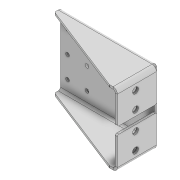
# Autodesk Inventor part: CCM_Mount_A
Saved by Autodesk Inventor 2020 (Build 240168000, 168)
## iProperties
Created: 2021-12-05
Part Number: CCM_Mount_A
Material: 一般
Document SubType Name: Sheet Metal
Designer: ken113
Density: 1 g/cm^3
Sheet Metal Rule: Default_mm
Appearance: 既定
Author: ken113
Autodesk Inventor part; units mm, degrees
ref_plane "YZ Plane" through (0, 0, 0) normal (1, 0, 0) x (0, 1, 0)
ref_plane "XZ Plane" through (0, 0, 0) normal (0, 1, 0) x (-1, 0, 0)
ref_plane "XY Plane" through (0, 0, 0) normal (0, 0, 1) x (1, 0, 0)
sketch "スケッチ1" plane through (0, 0, 0) normal (0, 0, 1) x (1, 0, 0)
  line L0 (-65, -50) -> (65, -50)
  line L1 (65, -50) -> (65, 50)
  line L2 (65, 50) -> (-65, 50)
  line L3 (-65, 50) -> (-65, -50)
  line L4 (-65, -50) -> (65, 50) construction
  line L5 (65, -50) -> (-65, 50) construction
  point P0 (0, 0)
  dimension "d0" = 130
  dimension "d1" = 100
  measures "d0" distance of L1.end L2.end
  measures "d1" distance of L2.end L0.start
extrude "プレート1" add sketch "スケッチ1" along normal blind 3
sketch "スケッチ2" plane through (-65, 47, 0) normal (0, 1, 0) x (-1, 0, 0)
  line L0 (-130, 0) -> (0, 0)
  line L1 (0, 0) -> (0, 60)
  line L2 (0, 60) -> (-130, 60)
  line L3 (-130, 60) -> (-130, 0)
  constraints: 6 end point, 1 horizontal, 1 perpendicular, 1 vertical
edge flange "フランジ1" height 60 angle 90 thickness 3 bend radius 3 thickness toward (0, 1, 0) relief straight relief width 3 relief depth 1.5 corner gap 3 corner form 0 edges at (0, 50, 3) (0, -50, 3) wall of the first edge with corners at (65, 47, 0) (-65, 47, 0) (-65, 47, 60) (65, 47, 60)
bend "曲げ1"
corner "コーナー1"
sketch "スケッチ3" plane through (68, 44, 60) normal (1, 0, 0) x (0, 1, 0)
  line L0 (0, -54) -> (0, 0)
  line L1 (0, 0) -> (-39, 0)
  line L2 (-39, 0) -> (-39, -54)
  line L3 (-39, -54) -> (0, -54)
  constraints: 6 end point, 1 horizontal, 1 perpendicular, 1 vertical
edge flange "フランジ2" height 45 angle 90 thickness 3 bend radius 3 thickness toward (1, 0, 0) relief straight relief width 3 relief depth 1.5 corner gap 3 corner form 0 edges at (65, 47, 33) (65, -47, 33) wall of the first edge with corners at (68, 44, 6) (68, 44, 60) (68, 5, 60) (68, 5, 6)
bend "曲げ2"
corner "コーナー2"
sketch "スケッチ4" plane through (-65, -50, 6) normal (0, -1, 0) x (1, 0, 0)
  line L0 (0, 0) -> (0, 54) projected
  line L1 (0, 5) -> (125, 54)
  line L2 (0, 54) -> (130, 54) projected
  line L3 (0, 0) -> (130, 0) projected
  line L4 (130, 54) -> (130, 0) projected
  point P0 (65, -6)
  dimension "d23" = 5
  dimension "d24" = 5
  constraints: 2 end point, 2 point on line
  measures "d23" distance from line of L1.start L3
  measures "d24" distance from line of L4 L1.end
extrude "押し出し1" cut sketch "スケッチ4" against normal through all contours L0 L2 L1
fillet "フィレット1" radius 2 8 edges at (-65, 48.5, 11) (-65, -48.5, 11) (60, 48.5, 60) (60, -48.5, 60) (69.5, 5, 60) (69.5, -5, 60) (69.5, 5, 6) (69.5, -5, 6)
sketch "スケッチ5" plane through (0, 0, 3) normal (0, 0, 1) x (1, 0, 0)
  line L0 (-55, -30) -> (-28, -30)
  line L1 (-28, -30) -> (-28, 30)
  line L2 (-28, 30) -> (-55, 30)
  line L3 (-55, 30) -> (-55, -30)
  line L4 (-55, -30) -> (-28, 30) construction
  line L5 (-28, -30) -> (-55, 30) construction
  line L6 (-65, -44) -> (-65, 44) projected
  point P0 (0, 0)
  point P1 (-41.5, 0)
  point P2 (-41.5, 0)
  point P3 (-55, 0)
  point P4 (-28, 0)
  dimension "d28" = 27
  dimension "d29" = 10
  dimension "d30" = 60
  constraints: 12 end point, 5 midpoint, 2 parallel, 1 horizontal, 1 horizontal alignment, 1 perpendicular
  measures "d28" distance of L1.end L2.end
  measures "d29" distance between parallel lines of L3 L6
  measures "d30" distance of L2.end L0.start
hole "穴1" at (-55, 0, 3) at (-28, 0, 3) at (-55, -30, 3) at (-55, 30, 3) at (-28, -30, 3) at (-28, 30, 3) direction (0, 0, -1) diameter 5.2 end through all
sketch "スケッチ6" plane through (68, 44, 6) normal (-1, 0, 0) x (0, 0, 1)
  arc A0 (0, -37) -> (2, -39) centre (2, -37) ccw projected
  line L0 (2, -39) -> (52, -39) projected
  arc A1 (52, -39) -> (54, -37) centre (52, -37) ccw projected
  line L1 (54, -37) -> (54, 0) projected
  line L2 (54, 0) -> (0, 0) projected
  line L3 (0, -37) -> (0, 0) projected
  arc A2 (2, -49) -> (0, -51) centre (2, -51) ccw projected
  line L4 (0, -51) -> (0, -88) projected
  line L5 (0, -88) -> (54, -88) projected
  line L6 (54, -51) -> (54, -88) projected
  arc A3 (54, -51) -> (52, -49) centre (52, -51) ccw projected
  line L7 (52, -49) -> (2, -49) projected
  point P0 (-6, -44)
  point P1 (29, -8)
  point P2 (29, -31)
  point P3 (29, -57)
  point P4 (29, -80)
  dimension "d38" = 25
  dimension "d39" = 8
  dimension "d40" = 8
  dimension "d41" = 8
  dimension "d42" = 8
  constraints: 3 vertical alignment
  measures "d38" distance from line of point (29, -80) L6
  measures "d39" distance from line of point (29, -80) L5
  measures "d40" distance from line of L7 point (29, -57)
  measures "d41" distance from line of point (29, -31) L0
  measures "d42" distance from line of L2 point (29, -8)
hole "穴2" at (68, 36, 35) at (68, 13, 35) at (68, -13, 35) at (68, -36, 35) direction (1, 0, 0) diameter 8.2 end through all
equation "\"d36\" = Thickness"
equation "\"d48\" = Thickness"
equation "\"d2\" = Thickness"
equation "\"d3\" = BendReliefWidth"
equation "\"d4\" = BendReliefDepth"
equation "\"d5\" = MinimumRemnant"
equation "\"d6\" = TransitionRadius"
equation "\"d9\" = BendRadius"
equation "\"d10\" = CornerReliefSize"
equation "\"d11\" = GapSize"
equation "\"d12\" = JacobiRadiusSize"
equation "\"d13\" = BendReliefWidth"
equation "\"d14\" = BendReliefDepth"
equation "\"d15\" = MinimumRemnant"
equation "\"d16\" = TransitionRadius"
equation "\"d19\" = BendRadius"
equation "\"d20\" = CornerReliefSize"
equation "\"d21\" = GapSize"
equation "\"d22\" = JacobiRadiusSize"
equation "\"BendRadius\" = Thickness"
equation "\"BendReliefWidth\" = Thickness"
equation "\"BendReliefDepth\" = 0.5 * Thickness"
equation "\"CornerReliefSize\" = 4 * Thickness"
equation "\"MinimumRemnant\" = 2 * Thickness"
equation "\"TransitionRadius\" = BendRadius"
equation "\"JacobiRadiusSize\" = BendRadius"
equation "\"GapSize\" = Thickness"
equation "\"Thickness\" = 3"
